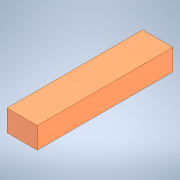
# Autodesk Inventor part: Contenedor3
Saved by Autodesk Inventor 2020.3 (Build 243373000, 373)
## iProperties
Created: 2020-09-22
Part Number: Contenedor3
Material: ABS Plastic
Document SubType Name: Modeling
Designer: juanp
Density: 1.06 g/cm^3
Appearance: Smooth - White
Author: juanp
Autodesk Inventor part; units mm, degrees
ref_plane "YZ Plane" through (0, 0, 0) normal (1, 0, 0) x (0, 1, 0)
sketch "Sketch1" plane through (0, 0, 0) normal (0, 1, 0) x (-1, 0, 0)
  line L0 (0, 0) -> (0, -358.09) construction
  line L1 (42, 13.0691) -> (0, 13.0691)
  line L2 (0, 13.0691) -> (0, -13.0691)
  line L3 (0, -13.0691) -> (42, -13.0691)
  line L4 (42, -13.0691) -> (42, 13.0691)
  line L5 (42, -15.0691) -> (0, -15.0691)
  line L6 (0, -15.0691) -> (0, -41.2074)
  line L7 (0, -41.2074) -> (42, -41.2074)
  line L8 (42, -41.2074) -> (42, -15.0691)
  line L9 (42, -43.2074) -> (0, -43.2074)
  line L10 (0, -43.2074) -> (0, -69.3457)
  line L11 (0, -69.3457) -> (42, -69.3457)
  line L12 (42, -69.3457) -> (42, -43.2074)
  line L13 (42, -101.4839) -> (0, -101.4839)
  line L14 (0, -101.4839) -> (0, -127.6222)
  line L15 (0, -127.6222) -> (42, -127.6222)
  line L16 (42, -127.6222) -> (42, -101.4839)
  line L17 (42, -129.6222) -> (0, -129.6222)
  line L18 (0, -129.6222) -> (0, -155.7604)
  line L19 (0, -155.7604) -> (42, -155.7604)
  line L20 (42, -155.7604) -> (42, -129.6222)
  line L21 (42, -73.3457) -> (0, -73.3457)
  line L22 (0, -73.3457) -> (0, -99.4839)
  line L23 (0, -99.4839) -> (42, -99.4839)
  line L24 (42, -99.4839) -> (42, -73.3457)
  line L25 (21, -13.0691) -> (21, -15.0691)
  line L26 (21, -41.2074) -> (21, -43.2074)
  line L27 (21, -99.4839) -> (21, -101.4839)
  line L28 (21, -127.6222) -> (21, -129.6222)
  line L29 (42, -159.7604) -> (0, -159.7604)
  line L30 (0, -159.7604) -> (0, -185.8987)
  line L31 (0, -185.8987) -> (42, -185.8987)
  line L32 (42, -185.8987) -> (42, -159.7604)
  line L33 (42, -187.8987) -> (0, -187.8987)
  line L34 (0, -187.8987) -> (0, -214.037)
  line L35 (0, -214.037) -> (42, -214.037)
  line L36 (42, -214.037) -> (42, -187.8987)
  line L37 (42, -216.037) -> (0, -216.037)
  line L38 (0, -216.037) -> (0, -242.1752)
  line L39 (0, -242.1752) -> (42, -242.1752)
  line L40 (42, -242.1752) -> (42, -216.037)
  line L41 (42, -274.3135) -> (0, -274.3135)
  line L42 (0, -274.3135) -> (0, -300.4517)
  line L43 (0, -300.4517) -> (42, -300.4517)
  line L44 (42, -300.4517) -> (42, -274.3135)
  line L45 (42, -302.4517) -> (0, -302.4517)
  line L46 (0, -302.4517) -> (0, -328.59)
  line L47 (0, -328.59) -> (42, -328.59)
  line L48 (42, -328.59) -> (42, -302.4517)
  line L49 (42, -246.1752) -> (0, -246.1752)
  line L50 (0, -246.1752) -> (0, -272.3135)
  line L51 (0, -272.3135) -> (42, -272.3135)
  line L52 (42, -272.3135) -> (42, -246.1752)
  line L53 (21, -185.8987) -> (21, -187.8987)
  line L54 (21, -214.037) -> (21, -216.037)
  line L55 (21, -272.3135) -> (21, -274.3135)
  line L56 (21, -300.4517) -> (21, -302.4517)
  line L57 (21, -328.59) -> (21, -330.59)
  line L58 (88, 15.0691) -> (-2, 15.0691)
  line L59 (-2, 15.0691) -> (-2, -387.59)
  line L60 (-2, -387.59) -> (88, -387.59)
  line L61 (88, -387.59) -> (88, 15.0691)
  line L62 (44, 0) -> (44, -358.09) construction
  line L63 (86, 13.0691) -> (44, 13.0691)
  line L64 (44, 13.0691) -> (44, -13.0691)
  line L65 (44, -13.0691) -> (86, -13.0691)
  line L66 (86, -13.0691) -> (86, 13.0691)
  line L67 (86, -15.0691) -> (44, -15.0691)
  line L68 (44, -15.0691) -> (44, -41.2074)
  line L69 (44, -41.2074) -> (86, -41.2074)
  line L70 (86, -41.2074) -> (86, -15.0691)
  line L71 (86, -43.2074) -> (44, -43.2074)
  line L72 (44, -43.2074) -> (44, -69.3457)
  line L73 (44, -69.3457) -> (86, -69.3457)
  line L74 (86, -69.3457) -> (86, -43.2074)
  line L75 (86, -101.4839) -> (44, -101.4839)
  line L76 (44, -101.4839) -> (44, -127.6222)
  line L77 (44, -127.6222) -> (86, -127.6222)
  line L78 (86, -127.6222) -> (86, -101.4839)
  line L79 (86, -129.6222) -> (44, -129.6222)
  line L80 (44, -129.6222) -> (44, -155.7604)
  line L81 (44, -155.7604) -> (86, -155.7604)
  line L82 (86, -155.7604) -> (86, -129.6222)
  line L83 (86, -73.3457) -> (44, -73.3457)
  line L84 (44, -73.3457) -> (44, -99.4839)
  line L85 (44, -99.4839) -> (86, -99.4839)
  line L86 (86, -99.4839) -> (86, -73.3457)
  line L87 (65, -13.0691) -> (65, -15.0691)
  line L88 (65, -41.2074) -> (65, -43.2074)
  line L89 (65, -99.4839) -> (65, -101.4839)
  line L90 (65, -127.6222) -> (65, -129.6222)
  line L91 (44, -216.037) -> (44, -242.1752)
  line L92 (86, -242.1752) -> (86, -216.037)
  line L93 (86, -246.1752) -> (44, -246.1752)
  line L94 (44, -246.1752) -> (44, -272.3135)
  line L95 (86, -272.3135) -> (86, -246.1752)
  line L96 (44, -242.1752) -> (86, -242.1752)
  line L97 (86, -159.7604) -> (44, -159.7604)
  line L98 (44, -159.7604) -> (44, -185.8987)
  line L99 (44, -185.8987) -> (86, -185.8987)
  line L100 (86, -185.8987) -> (86, -159.7604)
  line L101 (86, -216.037) -> (44, -216.037)
  line L102 (65, -214.037) -> (65, -216.037)
  line L103 (44, -214.037) -> (86, -214.037)
  line L104 (86, -214.037) -> (86, -187.8987)
  line L105 (86, -187.8987) -> (44, -187.8987)
  line L106 (44, -187.8987) -> (44, -214.037)
  line L107 (65, -185.8987) -> (65, -187.8987)
  line L108 (86, -274.3135) -> (44, -274.3135)
  line L109 (44, -274.3135) -> (44, -300.4517)
  line L110 (44, -300.4517) -> (86, -300.4517)
  line L111 (86, -300.4517) -> (86, -274.3135)
  line L112 (44, -272.3135) -> (86, -272.3135)
  line L113 (65, -300.4517) -> (65, -302.4517)
  line L114 (86, -302.4517) -> (44, -302.4517)
  line L115 (86, -328.59) -> (86, -302.4517)
  line L116 (44, -328.59) -> (86, -328.59)
  line L117 (44, -302.4517) -> (44, -328.59)
  line L118 (65, -272.3135) -> (65, -274.3135)
  line L119 (65, 13.0691) -> (65, 15.0691)
  line L120 (65, -69.3457) -> (65, -73.3457)
  line L121 (21, -69.3457) -> (21, -73.3457)
  line L122 (65, -155.7604) -> (65, -159.7604)
  line L123 (21, -155.7604) -> (21, -159.7604)
  line L124 (65, -242.1752) -> (65, -246.1752)
  line L125 (21, -242.1752) -> (21, -246.1752)
  line L126 (0, -330.59) -> (86, -330.59)
  line L127 (86, -330.59) -> (86, -385.59)
  line L128 (86, -385.59) -> (0, -385.59)
  line L129 (0, -385.59) -> (0, -330.59)
  line L130 (65, -328.59) -> (65, -330.59)
  line L131 (86, -358.09) -> (0, -358.09) construction
  point P0 (0, -28.1383)
  point P1 (0, -56.2765)
  point P2 (0, -114.553)
  point P3 (0, -142.6913)
  point P4 (0, -86.4148)
  point P5 (0, -172.8296)
  point P6 (0, -200.9678)
  point P7 (0, -229.1061)
  point P8 (0, -287.3826)
  point P9 (0, -315.5209)
  point P10 (0, -259.2443)
  point P11 (44, -28.1383)
  point P12 (44, -56.2765)
  point P13 (44, -114.553)
  point P14 (44, -142.6913)
  point P15 (44, -86.4148)
  point P16 (44, -229.1061)
  point P17 (44, -259.2443)
  point P18 (44, -172.8296)
  point P19 (44, -200.9678)
  point P20 (44, -287.3826)
  point P21 (44, -315.5209)
  point P22 (65, -244.1752)
  dimension "d0" = 358.09
  dimension "d7" = 2
  dimension "d8" = 2
  dimension "d10" = 358.09
  dimension "d12" = 2
  dimension "d13" = 2
  dimension "d14" = 90
  dimension "d15" = 2
  dimension "d16" = 4
  dimension "d17" = 4
  dimension "d18" = 4
  dimension "d24" = 2
  dimension "d25" = 55
  dimension "d26" = 402.6591
  dimension "d27" = 26.1383
  dimension "d28" = 86.4148
  constraints: 260 end point, 74 midpoint, 66 equal length, 52 parallel, 28 perpendicular, 26 horizontal, 4 point on line, 1 collinear, 1 vertical, 29 other
  measures "d0" distance of point (0, 0) point (0, -358.09)
  measures "d7" distance between parallel lines of L59 L2
  measures "d8" distance between parallel lines of L58 L1
  measures "d10" distance of point (44, 0) point (44, -358.09)
  measures "d12" distance of L119.start L119.end
  measures "d13" distance between parallel lines of L61 L74
  measures "d14" distance of L59.end L60.end
  measures "d15" distance between parallel lines of L4 L64
  measures "d16" distance of L121.start L121.end
  measures "d17" distance of L123.start L123.end
  measures "d18" distance of L125.start L125.end
  measures "d24" distance between parallel lines of L60 L128
  measures "d25" distance of L126.end L127.end
  measures "d26" distance between parallel lines of L60 L58
  measures "d27" distance of L48.start L45.start
  measures "d28" distance from line of point (65, -244.175) L126
extrude "Extrusion1" add sketch "Sketch1" along normal blind 60
sketch "Sketch2" plane through (0, 60, 0) normal (0, 1, 0) x (1, 0, 0)
  line L0 (2, -15.0691) -> (2, 387.59) projected
  line L1 (-88, -15.0691) -> (2, -15.0691) projected
  line L2 (-88, 387.59) -> (-88, -15.0691) projected
  line L3 (2, 387.59) -> (-88, 387.59) projected
  point P0 (0, 0)
extrude "Extrusion2" add sketch "Sketch2" along normal blind 3
fillet "Fillet1" radius 5 200 edges at (-42, 30, -43.2074) (0, 30, -43.2074) (-42, 30, -41.2074) (0, 30, -15.0691) (-21, 60, 13.0691) (-44, 30, -99.4839) (-44, 30, -101.4839) (-44, 30, -127.6222) (-86, 30, -127.6222) (-86, 30, -101.4839) (-86, 30, -73.3457) (0, 30, -69.3457) (-21, 60, -41.2074) (-86, 30, -13.0691) (-86, 30, -15.0691) (-44, 30, -15.0691) (-86, 30, 13.0691) (-44, 30, -13.0691) (-44, 30, 13.0691) (-42, 30, -15.0691) (-86, 60, -259.2443) (-42, 60, -287.3826) (-65, 60, -274.3135) (-86, 60, -287.3826) (-44, 60, -287.3826) (-42, 60, -259.2443) (-44, 60, -259.2443) (-42, 60, -229.1061) (-65, 60, -272.3135) (-65, 60, -300.4517) (0, 30, -41.2074) (-42, 60, -28.1383) (-21, 60, -15.0691) (-42, 30, -13.0691) (0, 30, -13.0691) (0, 30, 13.0691) (0, 30, -155.7604) (0, 30, -129.6222) (0, 30, -127.6222) (-42, 30, -155.7604) (-42, 30, -129.6222) (-86, 30, -129.6222) (-44, 30, -129.6222) (-86, 30, -155.7604) (-44, 30, -155.7604) (-86, 30, -159.7604) (-44, 60, -172.8296) (0, 30, -185.8987) (-42, 30, -159.7604) (-42, 30, -185.8987) (0, 30, -159.7604) (-44, 30, -41.2074) (-44, 30, -43.2074) (-44, 30, -69.3457) (-44, 30, -73.3457) (-86, 30, -41.2074) (-86, 30, -43.2074) (-21, 60, -13.0691) (-86, 30, -69.3457) (-42, 30, 13.0691) (-86, 30, -99.4839) (-65, 60, -214.037) (-86, 60, -200.9678) (-65, 60, -187.8987) (-44, 60, -200.9678) (-65, 60, -159.7604) (-65, 60, -185.8987) (-86, 60, -172.8296) (-65, 60, -155.7604) (-44, 30, -159.7604) (-86, 30, -185.8987) (-86, 30, -187.8987) (-86, 30, -214.037) (-44, 30, -214.037) (-44, 30, -185.8987) (0, 30, -214.037) (0, 30, -187.8987) (-42, 30, -187.8987) (-42, 30, -214.037) (-42, 60, -172.8296) (0, 60, -172.8296) (-21, 60, -187.8987) (-21, 60, -214.037) (-42, 60, -200.9678) (0, 60, -200.9678) (-21, 60, -216.037) (0, 60, -229.1061) (-21, 60, -185.8987) (-44, 30, -187.8987) (-86, 30, -216.037) (-44, 30, -216.037) (-86, 30, -242.1752) (-44, 30, -242.1752) (-86, 30, -246.1752) (-65, 60, -246.1752) (-65, 60, -242.1752) (-86, 60, -229.1061) (-44, 60, -229.1061) (-65, 60, -216.037) (0, 30, -242.1752) (0, 30, -216.037) (-42, 30, -242.1752) (-42, 30, -216.037) (-86, 30, -272.3135) (0, 30, -300.4517) (0, 30, -274.3135) (-42, 30, -274.3135) (-42, 30, -300.4517) (-44, 30, -246.1752) (-44, 30, -272.3135) (-44, 30, -274.3135) (-44, 30, -300.4517) (-86, 30, -300.4517) (-86, 30, -274.3135) (-42, 30, -302.4517) (-42, 30, -328.59) (0, 30, -302.4517) (-44, 30, -302.4517) (-86, 30, -302.4517) (-44, 30, -328.59) (-86, 30, -328.59) (0, 30, -328.59) (-21, 60, -242.1752) (-21, 60, -246.1752) (0, 60, -259.2443) (-21, 60, -272.3135) (0, 60, -287.3826) (-21, 60, -274.3135) (-21, 60, -300.4517) (-21, 60, -302.4517) (-65, 60, -302.4517) (-42, 60, -315.5209) (-21, 60, -328.59) (0, 60, -315.5209) (-44, 60, -315.5209) (-86, 60, -315.5209) (-65, 60, -328.59) (0, 30, -272.3135) (0, 30, -246.1752) (-42, 30, -246.1752) (-42, 30, -272.3135) (-65, 60, -69.3457) (-86, 60, -56.2765) (-65, 60, -43.2074) (-44, 60, -56.2765) (-65, 60, -41.2074) (-86, 60, -28.1383) (-65, 60, -15.0691) (-44, 60, -28.1383) (-65, 60, -13.0691) (-86, 60, 0) (-65, 60, 13.0691) (-44, 60, 0) (-44, 60, -142.6913) (-86, 60, -142.6913) (-65, 60, -127.6222) (-65, 60, -129.6222) (-86, 60, -114.553) (-44, 60, -114.553) (-65, 60, -101.4839) (-21, 60, -127.6222) (-21, 60, -129.6222) (0, 60, -142.6913) (-21, 60, -155.7604) (-42, 60, -142.6913) (-21, 60, -101.4839) (0, 60, -114.553) (-42, 60, -114.553) (-21, 60, -99.4839) (-21, 60, -73.3457) (-42, 60, -86.4148) (0, 60, -86.4148) (-21, 60, -159.7604) (-42, 30, -69.3457) (-42, 30, -127.6222) (0, 30, -101.4839) (-42, 30, -101.4839) (0, 30, -99.4839) (-42, 30, -99.4839) (-21, 60, -43.2074) (0, 60, -56.2765) (-42, 60, -56.2765) (-21, 60, -69.3457) (0, 60, -28.1383) (-42, 60, 0) (0, 60, 0) (0, 30, -73.3457) (-42, 30, -73.3457) (-86, 60, -86.4148) (-65, 60, -73.3457) (-44, 60, -86.4148) (-65, 60, -99.4839) (0, 30, -330.59) (0, 30, -385.59) (-86, 30, -385.59) (-86, 30, -330.59) (-43, 60, -330.59) (-86, 60, -358.09) (-43, 60, -385.59) (0, 60, -358.09)
ref_plane "Work Plane1" through (-88, 0, -186.2604) normal (0, 0, 1) x (1, 0, 0)
ref_plane "Work Plane2" through (-43, 0, 15.0691) normal (1, 0, 0) x (0, 0, -1)
body "Solid1"
